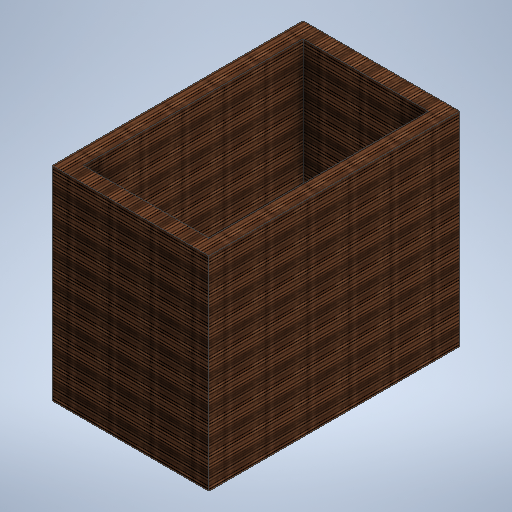
# Autodesk Inventor part: Caja
Saved by Autodesk Inventor 2025.2 (Build 292293000, 293)
## iProperties
Created: 2025-03-01
Part Number: Caja
Material: Genérico
Document SubType Name: Modeling
Designer: hmont
Density: 1 g/cm^3
Appearance: Valor por defecto
Author: hmont
Autodesk Inventor part; units mm, degrees
ref_plane "YZ Plane" through (0, 0, 0) normal (1, 0, 0) x (0, 1, 0)
ref_plane "XZ Plane" through (0, 0, 0) normal (0, 1, 0) x (-1, 0, 0)
ref_plane "XY Plane" through (0, 0, 0) normal (0, 0, 1) x (1, 0, 0)
sketch "Boceto1" plane through (0, 0, 0) normal (0, 1, 0) x (-1, 0, 0)
  line L0 (0, 0) -> (500, 0)
  line L1 (500, 0) -> (500, -800)
  line L2 (500, -800) -> (0, -800)
  line L3 (0, -800) -> (0, 0)
  line L4 (0, 0) -> (50, 0)
  line L5 (0, -50) -> (0, 0)
  line L6 (500, -800) -> (450, -800)
  line L7 (500, -750) -> (500, -800)
  line L8 (50, -50) -> (450, -50)
  line L9 (450, -50) -> (450, -750)
  line L10 (450, -750) -> (50, -750)
  line L11 (50, -750) -> (50, -50)
  dimension "d0" = 800
  dimension "d1" = 500
  dimension "d2" = 50
  dimension "d3" = 50
  constraints: 24 end point, 4 horizontal, 4 parallel, 2 perpendicular
  measures "d0" distance of L0.end L1.end
  measures "d1" distance of L1.end L2.end
  measures "d2" distance of L8.start L5.start
  measures "d3" distance of L4.end L8.start
extrude "Extrusión1" add sketch "Boceto1" along normal blind 600
sketch "Boceto2" plane through (0, 0, 0) normal (0, -1, 0) x (1, 0, 0)
  line L0 (0, -800) -> (-500, -800) projected
  line L1 (-500, -800) -> (0, -800)
  line L2 (0, -800) -> (0, 0)
  line L3 (0, 0) -> (-500, 0)
  line L4 (-500, 0) -> (-500, -800)
  constraints: 8 end point, 2 parallel, 1 horizontal, 1 perpendicular
extrude "Extrusión2" add sketch "Boceto2" along normal blind 50
